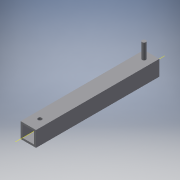
# Autodesk Inventor part: 1x1x8 Rectangular Tubing
Saved by Autodesk Inventor 2016 SP1 (Build 200210100, 210)
## iProperties
Created: 2016-01-21
Part Number: 1x1x8 Rectangular Tubing
Material: Generic
Document SubType Name: Modeling
Designer: steele
Density: 1 g/cm^3
Appearance: Default
Author: steele
Autodesk Inventor part; units mm, degrees
ref_plane "YZ Plane" through (0, 0, 0) normal (1, 0, 0) x (0, 1, 0)
ref_plane "XZ Plane" through (0, 0, 0) normal (0, 1, 0) x (-1, 0, 0)
ref_plane "XY Plane" through (0, 0, 0) normal (0, 0, 1) x (1, 0, 0)
sketch "Sketch1" plane through (0, 0, 0) normal (0, 0, 1) x (1, 0, 0)
  line L0 (-12.7, -12.7) -> (12.7, -12.7)
  line L1 (12.7, -12.7) -> (12.7, 12.7)
  line L2 (12.7, 12.7) -> (-12.7, 12.7)
  line L3 (-12.7, 12.7) -> (-12.7, -12.7)
  line L4 (-12.7, -12.7) -> (12.7, 12.7) construction
  line L5 (12.7, -12.7) -> (-12.7, 12.7) construction
  line L6 (-9.525, -9.525) -> (9.525, -9.525)
  line L7 (9.525, -9.525) -> (9.525, 9.525)
  line L8 (9.525, 9.525) -> (-9.525, 9.525)
  line L9 (-9.525, 9.525) -> (-9.525, -9.525)
  line L10 (-9.525, -9.525) -> (9.525, 9.525) construction
  line L11 (9.525, -9.525) -> (-9.525, 9.525) construction
  point P0 (0, 0)
  dimension "d0" = 3.175
  dimension "d1" = 25.4
  constraints: 24 end point, 4 midpoint, 4 parallel, 4 perpendicular, 2 horizontal
  measures "d0" distance between parallel lines of L9 L3
  measures "d1" distance of L2.end L0.start
extrude "Extrusion1" add sketch "Sketch1" along normal mid plane 203.2
sketch "Sketch2" plane through (-12.7, 12.7, 101.6) normal (0, 1, 0) x (1, 0, 0)
  line L0 (0, 203.2) -> (25.4, 203.2) construction
  line L1 (12.7, 203.2) -> (12.7, 0) construction
  line L2 (22.225, 0) -> (3.175, 0) construction
  circle A0 centre (12.7, 19.05) radius 3.175
  line L3 (25.4, 0) -> (0, 0) projected
  point P0 (12.7, 101.6)
  dimension "d4" = 6.35
  dimension "d5" = 19.05
  constraints: 2 end point, 2 midpoint, 1 centre point, 1 point on line
  measures "d4" diameter of A0
  measures "d5" distance from line of A0.centre L3
extrude "Extrusion2" cut sketch "Sketch2" against normal through all
sketch "Sketch3" plane through (-12.7, 12.7, 101.6) normal (0, 1, 0) x (1, 0, 0)
  line L0 (0, 203.2) -> (25.4, 203.2) construction
  line L1 (12.7, 203.2) -> (12.7, 0) construction
  line L2 (25.4, 0) -> (0, 0) construction
  circle A0 centre (12.7, 190.5) radius 3.175
  point P0 (12.7, 101.6)
  dimension "d8" = 6.35
  dimension "d9" = 12.7
  constraints: 2 end point, 2 midpoint, 1 centre point, 1 point on line
  measures "d8" diameter of A0
  measures "d9" distance from line of A0.centre L0
extrude "Extrusion3" add sketch "Sketch3" along normal blind 25.4
body "Solid1"
